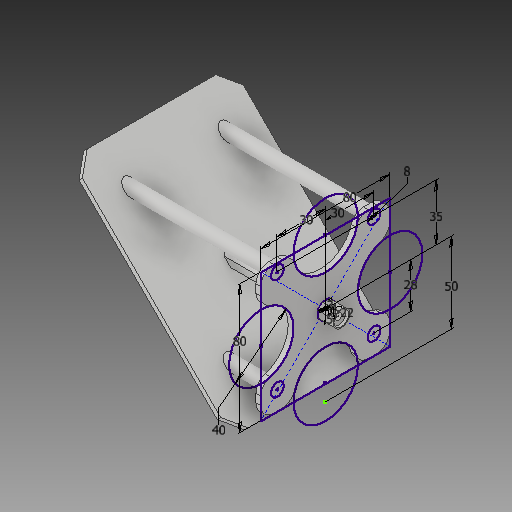
# Autodesk Inventor part: MIRROR MOUNT
Saved by Autodesk Inventor 2017 (Build 210142000, 142)
## iProperties
Created: 2017-04-01
Part Number: MIRROR MOUNT
Material: Generic
Document SubType Name: Modeling
Designer: Muchen
Density: 1 g/cm^3
Appearance: Default
Mass: 69.4214 g
Surface Area: 451.287 cm^2
Volume: 69.4214 cm^3
Author: Muchen
Autodesk Inventor part; units mm, degrees
ref_plane "YZ Plane" through (0, 0, 0) normal (1, 0, 0) x (0, 1, 0)
ref_plane "XZ Plane" through (0, 0, 0) normal (0, 1, 0) x (-1, 0, 0)
ref_plane "XY Plane" through (0, 0, 0) normal (0, 0, 1) x (1, 0, 0)
sketch "Sketch1" plane through (0, 0, 0) normal (0, 0, 1) x (1, 0, 0)
  line L0 (-10, 0) -> (-7.8787, 2.1213)
  line L1 (-7.8787, 2.1213) -> (-107.8787, 102.1213)
  line L2 (-107.8787, 102.1213) -> (-110, 100)
  line L3 (-110, 100) -> (-10, 0)
  line L4 (-10, 0) -> (0, 0) construction
  dimension "d24" = 10
  dimension "d25" = 3
  dimension "d26" = 45
  dimension "d27" = 100
  constraints: 10 end point, 2 parallel, 1 horizontal, 1 perpendicular
  measures "d24" distance of L0.start L4.end
  measures "d25" distance of L0.start L0.end
  measures "d26" angle of L4 L0
  measures "d27" horizontal distance of L2.end L0.start
extrude "Extrusion1" add sketch "Sketch1" along normal mid plane 100
chamfer "Chamfer1" distance 10 angle 45 4 edges at (-108.9393, 101.0607, 50) (-8.9393, 1.0607, 50) (-8.9393, 1.0607, -50) (-108.9393, 101.0607, -50)
sketch "Sketch2" plane through (0, 0, 0) normal (1, 0, 0) x (0, 1, 0)
  arc A0 (51.5, -1.3229) -> (51.5, 1.3229) centre (50, 0) ccw
  line L0 (55, -2.0711) -> (52.0711, -5)
  line L1 (52.0711, -5) -> (47.9289, -5)
  line L2 (47.9289, -5) -> (45, -2.0711)
  line L3 (45, -2.0711) -> (45, 2.0711)
  line L4 (45, 2.0711) -> (47.9289, 5)
  line L5 (47.9289, 5) -> (52.0711, 5)
  line L6 (52.0711, 5) -> (55, 2.0711)
  line L7 (55, 2.0711) -> (55, -2.0711)
  line L8 (51.5, 1.3229) -> (51.5, -1.3229)
  line L9 (48.5, 1.3229) -> (48.5, -1.3229)
  arc A1 (48.5, -1.3229) -> (51.5, -1.3229) centre (50, 0) ccw
  arc A2 (51.5, 1.3229) -> (48.5, -1.3229) centre (50, 0) ccw
  circle A3 centre (85, 30) radius 4
  circle A4 centre (85, -30) radius 4
  circle A5 centre (22, 30) radius 4
  circle A6 centre (22, -30) radius 4
  line L10 (10, 40) -> (90, 40)
  line L11 (90, 40) -> (90, -40)
  line L12 (90, -40) -> (10, -40)
  line L13 (10, -40) -> (10, 40)
  line L14 (10, 40) -> (90, -40) construction
  line L15 (90, 40) -> (10, -40) construction
  circle A7 centre (50, 40) radius 20
  circle A8 centre (50, -40) radius 20
  circle A9 centre (90, 0) radius 20
  circle A10 centre (50, 0) radius 4.61
  circle A11 centre (10, 0) radius 20
  point P0 (0, 0)
  point P1 (0, 0)
  point P2 (50, 0)
  dimension "d8" = 50
  dimension "d10" = 4
  dimension "d11" = 5
  dimension "d14" = 3
  dimension "d15" = 30
  dimension "d16" = 30
  dimension "d17" = 35
  dimension "d18" = 28
  dimension "d19" = 8
  dimension "d28" = 80
  dimension "d29" = 80
  dimension "d35" = 9.22
  dimension "d38" = 40
  constraints: 32 end point, 12 centre point, 8 point on circle, 7 coincident, 7 midpoint, 6 equal radius, 4 horizontal alignment, 3 parallel, 3 vertical alignment, 2 horizontal, 2 vertical, 1 perpendicular, 17 other
  measures "d8" distance of point (0, 0) point (50, 0)
  measures "d10" diameter of A0
  measures "d11" distance from line of point (50, 0) L1
  measures "d14" distance between parallel lines of L8 L9
  measures "d15" vertical distance of point (50, 0) A3.centre
  measures "d16" vertical distance of point (50, 0) A4.centre
  measures "d17" horizontal distance of point (50, 0) A3.centre
  measures "d18" horizontal distance of A6.centre point (50, 0)
  measures "d19" diameter of A4
  measures "d28" distance of L10.end L11.end
  measures "d29" distance of L10.start L10.end
  measures "d35" diameter of A10
  measures "d38" diameter of A7
extrude "Extrusion2" add sketch "Sketch2" against normal up to next contours L8 A0 | A1 L9 A2 L8 | A2 L9 | L0 L1 L2 L3 L4 L5 L6 L7 | A10
extrude "Extrusion3" add sketch "Sketch2" against normal blind 3 contours A7 L10 | L10 L11 A9 L12 A8 L13 A11 A7 | L11 A9 | A11 L13 | L12 A8 picked at (44.8162, 33.9837) picked at (86.9018, -5.903) picked at (22.2846, 1.4835) picked at (43.3333, -31.1584)
extrude "Extrusion4" add sketch "Sketch2" against normal up to next contours A3 | A4 | A5 | A6
extrude "Extrusion5" cut sketch "Sketch2" against normal up to surface (3 mm away) contours A7 L10 | L10 A7 | A9 L11 | L11 A9 | A11 L13 | L13 A11 | A8 L12 | L12 A8
fillet "Fillet2" radius 8 12 edges at (-1.5, 30, 40) (-1.5, 70, 40) (-1.5, 10, 40) (-1.5, 10, -40) (-1.5, 70, -40) (-1.5, 30, -40) (-1.5, 90, -40) (-1.5, 90, 20) (-1.5, 90, -20) (-1.5, 90, 40) (-1.5, 10, 20) (-1.5, 10, -20)
extrude "Extrusion7" add sketch "Sketch2" along normal blind 10 contours L0 L1 L2 L3 L4 L5 L6 L7
extrude "Extrusion8" add sketch "Sketch2" along normal blind 8.25 contours A10
extrude "Extrusion9" add sketch "Sketch2" along normal blind 6.22 contours L8 A0 | A2 L9
body "Solid1"
